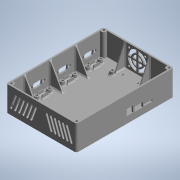
# Autodesk Inventor part: skr_case
Saved by Autodesk Inventor 2022 (Build 260153000, 153)
## iProperties
Part Number: skr_case
Material: Allgemein
Document SubType Name: Modellieren
Designer: Niclas
Appearance: Vorgabe
Author: Niclas
Autodesk Inventor part; units mm, degrees
ref_plane "YZ-Ebene" through (0, 0, 0) normal (1, 0, 0) x (0, 1, 0)
ref_plane "XZ-Ebene" through (0, 0, 0) normal (0, 1, 0) x (-1, 0, 0)
ref_plane "XY-Ebene" through (0, 0, 0) normal (0, 0, 1) x (1, 0, 0)
sketch "Skizze1" plane through (0, 0, 0) normal (0, 1, 0) x (-1, 0, 0)
  line L0 (0, 0) -> (-140, 0)
  line L1 (-140, 0) -> (-140, -194)
  line L2 (-140, -194) -> (0, -194)
  line L3 (0, -194) -> (0, 0)
  dimension "d0" = 194
  dimension "d1" = 140
  constraints: 8 end point, 2 parallel, 1 coincident, 1 horizontal, 1 perpendicular
  measures "d0" distance of L2.end L0.start
  measures "d1" distance of L0.start L0.end
extrude "Extrusion1" add sketch "Skizze1" along normal blind 5
sketch "Skizze2" plane through (0, 5, 0) normal (0, 1, 0) x (1, 0, 0)
  circle A0 centre (45, 28) radius 4
  circle A1 centre (45, 166) radius 4
  circle A2 centre (132, 28) radius 4
  circle A3 centre (132, 166) radius 4
  line L0 (140, 0) -> (140, 194) projected
  line L1 (140, 194) -> (0, 194) projected
  circle A4 centre (45, 28) radius 2.25
  circle A5 centre (132, 28) radius 2.25
  circle A6 centre (132, 166) radius 2.25
  circle A7 centre (45, 166) radius 2.25
  point P0 (0, 0)
  dimension "d4" = 138
  dimension "d5" = 138
  dimension "d6" = 87
  dimension "d7" = 87
  dimension "d8" = 8
  dimension "d9" = 8
  dimension "d10" = 8
  dimension "d11" = 8
  dimension "d12" = 8
  dimension "d13" = 8
  dimension "d14" = 28
  dimension "d15" = 28
  dimension "d16" = 4.5
  dimension "d17" = 4.5
  dimension "d18" = 4.5
  dimension "d19" = 4.5
  constraints: 8 centre point, 4 coincident
  measures "d4" distance of A3.centre A2.centre
  measures "d5" distance of A1.centre A0.centre
  measures "d6" distance of A2.centre A0.centre
  measures "d7" distance of A3.centre A1.centre
  measures "d8" distance from line of L0 A2.centre
  measures "d9" distance from line of L0 A3.centre
  measures "d10" diameter of A2
  measures "d11" diameter of A3
  measures "d12" diameter of A1
  measures "d13" diameter of A0
  measures "d14" distance from line of L1 A3.centre
  measures "d15" distance from line of L1 A1.centre
  measures "d16" diameter of A4
  measures "d17" diameter of A5
  measures "d18" diameter of A6
  measures "d19" diameter of A7
extrude "Extrusion2" add sketch "Skizze2" along normal blind 7
chamfer "Fase1" distance 2 angle 45 4 edges at (128, 5, -28) (41, 5, -28) (41, 5, -166) (128, 5, -166)
sketch "Skizze3" plane through (0, 5, 0) normal (0, 1, 0) x (1, 0, 0)
  line L0 (3, 3) -> (137, 3)
  line L1 (137, 3) -> (137, 191)
  line L2 (137, 191) -> (3, 191)
  line L3 (3, 191) -> (3, 3)
  line L4 (0, 194) -> (0, 0) projected
  line L5 (0, 0) -> (140, 0) projected
  line L6 (140, 0) -> (140, 194) projected
  line L7 (140, 194) -> (0, 194) projected
  line L8 (0, 0) -> (140, 0)
  line L9 (140, 0) -> (140, 194)
  line L10 (140, 194) -> (0, 194)
  line L11 (0, 194) -> (0, 0)
  dimension "d25" = 3
  dimension "d26" = 3
  dimension "d27" = 3
  dimension "d28" = 3
  constraints: 16 end point, 4 parallel, 2 horizontal, 2 perpendicular
  measures "d25" distance between parallel lines of L3 L4
  measures "d26" distance between parallel lines of L5 L0
  measures "d27" distance between parallel lines of L6 L1
  measures "d28" distance between parallel lines of L7 L2
extrude "Extrusion3" add sketch "Skizze3" along normal blind 45
sketch "Skizze4" plane through (140, 0, 0) normal (1, 0, 0) x (0, 0, -1)
  line L0 (99.85, 25.4) -> (112.85, 25.4)
  line L1 (112.85, 25.4) -> (112.85, 13.4)
  line L2 (112.85, 13.4) -> (99.85, 13.4)
  line L3 (99.85, 13.4) -> (99.85, 25.4)
  line L4 (0, 0) -> (194, 0) projected
  line L5 (194, 0) -> (194, 50) projected
  line L6 (115.9, 21.6) -> (132.4, 21.6)
  line L7 (132.4, 21.6) -> (132.4, 12.6)
  line L8 (132.4, 12.6) -> (115.9, 12.6)
  line L9 (115.9, 12.6) -> (115.9, 21.6)
  line L10 (134.15, 16.8) -> (151.15, 16.8)
  line L11 (151.15, 16.8) -> (151.15, 13.3)
  line L12 (151.15, 13.3) -> (134.15, 13.3)
  line L13 (134.15, 13.3) -> (134.15, 16.8)
  dimension "d31" = 12
  dimension "d32" = 13
  dimension "d33" = 13.4
  dimension "d34" = 81.15
  dimension "d37" = 9
  dimension "d38" = 16.5
  dimension "d39" = 61.6
  dimension "d40" = 12.6
  dimension "d41" = 17
  dimension "d42" = 3.5
  dimension "d43" = 42.85
  dimension "d44" = 13.3
  constraints: 24 end point, 6 parallel, 3 horizontal, 3 perpendicular
  measures "d31" distance of L0.end L1.end
  measures "d32" distance of L1.end L2.end
  measures "d33" distance between parallel lines of L4 L2
  measures "d34" distance between parallel lines of L5 L1
  measures "d37" distance of L6.end L7.end
  measures "d38" distance of L7.end L8.end
  measures "d39" distance between parallel lines of L5 L7
  measures "d40" distance between parallel lines of L4 L8
  measures "d41" distance of L10.start L10.end
  measures "d42" distance of L10.end L11.end
  measures "d43" distance between parallel lines of L5 L11
  measures "d44" distance between parallel lines of L4 L12
extrude "Extrusion4" cut sketch "Skizze4" against normal blind 40
sketch "Skizze5" plane through (0, 0, -194) normal (-1, 0, 0) x (0, 0, 1)
  line L0 (128.4836, 25) -> (140.5164, 25)
  line L1 (143.4832, 21.555) -> (142.8832, 17.555)
  line L2 (139.9164, 15) -> (129.0836, 15)
  line L3 (126.1168, 17.555) -> (125.5168, 21.555)
  arc A0 (128.4836, 25) -> (125.5168, 21.555) centre (128.4836, 22) ccw
  arc A1 (126.1168, 17.555) -> (129.0836, 15) centre (129.0836, 18) ccw
  arc A2 (139.9164, 15) -> (142.8832, 17.555) centre (139.9164, 18) ccw
  arc A3 (143.4832, 21.555) -> (140.5164, 25) centre (140.5164, 22) ccw
  circle A4 centre (122, 20) radius 2.75
  circle A5 centre (147, 20) radius 2.75
  line L4 (77.4836, 25) -> (89.5164, 25)
  line L5 (92.4832, 21.555) -> (91.8832, 17.555)
  line L6 (88.9164, 15) -> (78.0836, 15)
  line L7 (75.1168, 17.555) -> (74.5168, 21.555)
  arc A6 (77.4836, 25) -> (74.5168, 21.555) centre (77.4836, 22) ccw
  arc A7 (75.1168, 17.555) -> (78.0836, 15) centre (78.0836, 18) ccw
  arc A8 (88.9164, 15) -> (91.8832, 17.555) centre (88.9164, 18) ccw
  arc A9 (92.4832, 21.555) -> (89.5164, 25) centre (89.5164, 22) ccw
  circle A10 centre (71, 20) radius 2.75
  circle A11 centre (96, 20) radius 2.75
  line L8 (26.4836, 25) -> (38.5164, 25)
  line L9 (41.4832, 21.555) -> (40.8832, 17.555)
  line L10 (37.9164, 15) -> (27.0836, 15)
  line L11 (24.1168, 17.555) -> (23.5168, 21.555)
  arc A12 (26.4836, 25) -> (23.5168, 21.555) centre (26.4836, 22) ccw
  arc A13 (24.1168, 17.555) -> (27.0836, 15) centre (27.0836, 18) ccw
  arc A14 (37.9164, 15) -> (40.8832, 17.555) centre (37.9164, 18) ccw
  arc A15 (41.4832, 21.555) -> (38.5164, 25) centre (38.5164, 22) ccw
  circle A16 centre (20, 20) radius 2.75
  circle A17 centre (45, 20) radius 2.75
  line L12 (0, 50) -> (194, 50) projected
  line L13 (0, 0) -> (0, 50) projected
  circle A18 centre (172.5, 20) radius 4
  line L14 (0, 0) -> (194, 0) projected
  point P0 (125, 25)
  point P1 (144, 25)
  point P2 (142.5, 15)
  point P3 (126.5, 15)
  point P4 (74, 25)
  point P5 (93, 25)
  point P6 (91.5, 15)
  point P7 (75.5, 15)
  point P8 (23, 25)
  point P9 (42, 25)
  point P10 (40.5, 15)
  point P11 (24.5, 15)
  dimension "d45" = 19
  dimension "d46" = 16
  dimension "d47" = 10
  dimension "d48" = 1.5
  dimension "d49" = 3
  dimension "d50" = 25
  dimension "d51" = 5.5
  dimension "d52" = 5.5
  dimension "d53" = 5
  dimension "d54" = 5
  dimension "d55" = 4.5
  dimension "d56" = 19
  dimension "d57" = 16
  dimension "d58" = 10
  dimension "d59" = 1.5
  dimension "d60" = 3
  dimension "d61" = 25
  dimension "d62" = 5.5
  dimension "d63" = 5.5
  dimension "d64" = 5
  dimension "d65" = 5
  dimension "d66" = 4.5
  dimension "d67" = 19
  dimension "d68" = 16
  dimension "d69" = 10
  dimension "d70" = 1.5
  dimension "d71" = 3
  dimension "d72" = 25
  dimension "d73" = 5.5
  dimension "d74" = 5.5
  dimension "d75" = 5
  dimension "d76" = 5
  dimension "d77" = 4.5
  dimension "d142" = 20
  dimension "d143" = 26
  dimension "d144" = 26
  dimension "d145" = 8
  dimension "d146" = 25.5
  dimension "d147" = 0
  dimension "d267" = 20
  dimension "d268" = 20
  dimension "d269" = 20
  constraints: 24 end point, 24 point on circle, 24 point on line, 24 tangent, 19 centre point, 9 equal radius, 3 horizontal, 3 parallel
  measures "d45" distance of point (125, 25) point (144, 25)
  measures "d46" distance of point (142.5, 15) point (126.5, 15)
  measures "d47" vertical distance of point (126.5, 15) point (125, 25)
  measures "d48" horizontal distance of point (125, 25) point (126.5, 15)
  measures "d49" radius of A0
  measures "d50" distance of A5.centre A4.centre
  measures "d51" diameter of A5
  measures "d52" diameter of A4
  measures "d53" vertical distance of point (142.5, 15) A5.centre
  measures "d54" vertical distance of point (126.5, 15) A4.centre
  measures "d55" horizontal distance of point (142.5, 15) A5.centre
  measures "d56" distance of point (74, 25) point (93, 25)
  measures "d57" distance of point (91.5, 15) point (75.5, 15)
  measures "d58" vertical distance of point (75.5, 15) point (74, 25)
  measures "d59" horizontal distance of point (74, 25) point (75.5, 15)
  measures "d60" radius of A6
  measures "d61" distance of A11.centre A10.centre
  measures "d62" diameter of A11
  measures "d63" diameter of A10
  measures "d64" vertical distance of point (91.5, 15) A11.centre
  measures "d65" vertical distance of point (75.5, 15) A10.centre
  measures "d66" horizontal distance of point (91.5, 15) A11.centre
  measures "d67" distance of point (23, 25) point (42, 25)
  measures "d68" distance of point (40.5, 15) point (24.5, 15)
  measures "d69" vertical distance of point (24.5, 15) point (23, 25)
  measures "d70" horizontal distance of point (23, 25) point (24.5, 15)
  measures "d71" radius of A12
  measures "d72" distance of A17.centre A16.centre
  measures "d73" diameter of A17
  measures "d74" diameter of A16
  measures "d75" vertical distance of point (40.5, 15) A17.centre
  measures "d76" vertical distance of point (24.5, 15) A16.centre
  measures "d77" horizontal distance of point (40.5, 15) A17.centre
  measures "d142" distance from line of L13 A16.centre
  measures "d143" distance of A17.centre A10.centre
  measures "d144" distance of A11.centre A4.centre
  measures "d145" diameter of A18
  measures "d146" distance of A5.centre A18.centre
  measures "d147" vertical distance of A5.centre A18.centre
  measures "d267" distance from line of L14 A16.centre
  measures "d268" distance from line of L14 A10.centre
  measures "d269" distance from line of L14 A4.centre
extrude "Extrusion5" cut sketch "Skizze5" against normal blind 40
sketch "Skizze6" plane through (0, 5, 0) normal (0, 1, 0) x (1, 0, 0)
  circle A0 centre (13.5, 149) radius 4
  circle A1 centre (13.5, 174) radius 4
  circle A2 centre (13.5, 149) radius 2.25
  circle A3 centre (13.5, 174) radius 2.25
  line L0 (140, 194) -> (0, 194) projected
  line L1 (0, 194) -> (0, 0) projected
  line L2 (8.5, 155.5) -> (9.5, 155.5)
  line L3 (9.5, 155.5) -> (9.5, 167.5)
  line L4 (9.5, 167.5) -> (8.5, 167.5)
  line L5 (8.5, 167.5) -> (8.5, 155.5)
  line L6 (17.5, 155.5) -> (18.5, 155.5)
  line L7 (18.5, 155.5) -> (18.5, 167.5)
  line L8 (18.5, 167.5) -> (17.5, 167.5)
  line L9 (17.5, 167.5) -> (17.5, 155.5)
  circle A4 centre (13.5, 98) radius 4
  circle A5 centre (13.5, 123) radius 4
  circle A6 centre (13.5, 98) radius 2.25
  circle A7 centre (13.5, 123) radius 2
  line L10 (8.5, 104.5) -> (9.5, 104.5)
  line L11 (9.5, 104.5) -> (9.5, 116.5)
  line L12 (9.5, 116.5) -> (8.5, 116.5)
  line L13 (8.5, 116.5) -> (8.5, 104.5)
  line L14 (17.5, 104.5) -> (18.5, 104.5)
  line L15 (18.5, 104.5) -> (18.5, 116.5)
  line L16 (18.5, 116.5) -> (17.5, 116.5)
  line L17 (17.5, 116.5) -> (17.5, 104.5)
  line L18 (17.5, 53.5) -> (18.5, 53.5)
  line L19 (18.5, 53.5) -> (18.5, 65.5)
  line L20 (17.5, 65.5) -> (17.5, 53.5)
  line L21 (8.5, 53.5) -> (9.5, 53.5)
  line L22 (9.5, 53.5) -> (9.5, 65.5)
  line L23 (8.5, 65.5) -> (8.5, 53.5)
  circle A8 centre (13.5, 47) radius 2.25
  circle A9 centre (13.5, 47) radius 4
  circle A10 centre (13.5, 72) radius 4
  circle A11 centre (13.5, 72) radius 2.25
  line L24 (9.5, 65.5) -> (8.5, 65.5)
  line L25 (18.5, 65.5) -> (17.5, 65.5)
  line L26 (3, 3) -> (3, 191) projected
  dimension "d86" = 8
  dimension "d87" = 8
  dimension "d88" = 25
  dimension "d89" = 4.5
  dimension "d90" = 4.5
  dimension "d91" = 20
  dimension "d94" = 1
  dimension "d95" = 12
  dimension "d96" = 12
  dimension "d97" = 1
  dimension "d98" = 4
  dimension "d99" = 4
  dimension "d100" = 6.5
  dimension "d101" = 8
  dimension "d102" = 8
  dimension "d103" = 25
  dimension "d104" = 4.5
  dimension "d105" = 4
  dimension "d106" = 1
  dimension "d107" = 12
  dimension "d108" = 12
  dimension "d109" = 1
  dimension "d110" = 4
  dimension "d111" = 4
  dimension "d112" = 6.5
  dimension "d113" = 26
  dimension "d116" = 8
  dimension "d117" = 8
  dimension "d118" = 25
  dimension "d119" = 4.5
  dimension "d120" = 4.5
  dimension "d121" = 1
  dimension "d122" = 12
  dimension "d123" = 12
  dimension "d124" = 1
  dimension "d125" = 4
  dimension "d126" = 4
  dimension "d127" = 6.5
  dimension "d128" = 26
  dimension "d131" = 10.5
  dimension "d132" = 10.5
  dimension "d133" = 10.5
  dimension "d134" = 10.5
  dimension "d135" = 10.5
  dimension "d136" = 10.5
  constraints: 48 end point, 12 centre point, 12 parallel, 6 coincident, 6 horizontal, 6 perpendicular, 3 point on line
  measures "d86" diameter of A1
  measures "d87" diameter of A0
  measures "d88" distance of A1.centre A0.centre
  measures "d89" diameter of A2
  measures "d90" diameter of A3
  measures "d91" distance from line of L0 A1.centre
  measures "d94" distance of L2.start L2.end
  measures "d95" distance of L4.end L2.start
  measures "d96" distance of L8.end L6.start
  measures "d97" distance of L6.start L6.end
  measures "d98" distance from line of L9 A0.centre
  measures "d99" distance from line of L3 A0.centre
  measures "d100" vertical distance of A0.centre L2.end
  measures "d101" diameter of A5
  measures "d102" diameter of A4
  measures "d103" distance of A5.centre A4.centre
  measures "d104" diameter of A6
  measures "d105" diameter of A7
  measures "d106" distance of L10.start L10.end
  measures "d107" distance of L13.start L10.start
  measures "d108" distance of L17.start L14.start
  measures "d109" distance of L14.start L14.end
  measures "d110" distance from line of L17 A4.centre
  measures "d111" distance from line of L11 A4.centre
  measures "d112" vertical distance of A4.centre L10.end
  measures "d113" distance of A7.centre A0.centre
  measures "d116" diameter of A10
  measures "d117" diameter of A9
  measures "d118" distance of A10.centre A9.centre
  measures "d119" diameter of A8
  measures "d120" diameter of A11
  measures "d121" distance of L21.start L22.start
  measures "d122" distance of L24.end L21.start
  measures "d123" distance of L25.end L18.start
  measures "d124" distance of L18.start L19.start
  measures "d125" distance from line of L20 A9.centre
  measures "d126" distance from line of L22 A9.centre
  measures "d127" vertical distance of A9.centre L22.start
  measures "d128" distance of A4.centre A11.centre
  measures "d131" distance from line of L26 A9.centre
  measures "d132" distance from line of L26 A11.centre
  measures "d133" distance from line of L26 A6.centre
  measures "d134" distance from line of L26 A5.centre
  measures "d135" distance from line of L26 A0.centre
  measures "d136" distance from line of L26 A1.centre
extrude "Extrusion6" add sketch "Skizze6" along normal blind 7.5
chamfer "Fase2" distance 2 angle 45 30 edges at (9.5, 5, -47) (9.5, 5, -72) (9.5, 5, -98) (9.5, 5, -123) (9.5, 5, -149) (9.5, 5, -174) (18.5, 5, -161.5) (18.5, 5, -110.5) (18.5, 5, -59.5) (9.5, 5, -110.5) (9.5, 5, -161.5) (9.5, 5, -59.5) (18, 5, -104.5) (18, 5, -53.5) (18, 5, -155.5) (9, 5, -53.5) (9, 5, -104.5) (9, 5, -155.5) (18, 5, -65.5) (18, 5, -116.5) (18, 5, -167.5) (9, 5, -167.5) (9, 5, -116.5) (9, 5, -65.5) (8.5, 5, -161.5) (8.5, 5, -110.5) (8.5, 5, -59.5) (17.5, 5, -59.5) (17.5, 5, -110.5) (17.5, 5, -161.5)
sketch "Skizze7" plane through (3, 5, -3) normal (1, 0, 0) x (0, 0, -1)
  line L0 (132, 0) -> (134, 0)
  line L1 (134, 0) -> (134, 45)
  line L2 (134, 45) -> (132, 45)
  line L3 (132, 45) -> (132, 0)
  circle A0 centre (120, 15) radius 2.75 projected
  line L4 (81, 0) -> (83, 0)
  line L5 (83, 0) -> (83, 45)
  line L6 (83, 45) -> (81, 45)
  line L7 (81, 45) -> (81, 0)
  circle A1 centre (69, 15) radius 2.75 projected
  line L8 (32, 0) -> (30, 0)
  line L9 (30, 0) -> (30, 45)
  line L10 (30, 45) -> (32, 45)
  line L11 (32, 45) -> (32, 0)
  circle A2 centre (18.5, 15) radius 4 projected
  circle A3 centre (171, 15) radius 2.75 projected
  circle A4 centre (146, 15) radius 2.75 projected
  circle A5 centre (95, 15) radius 2.75 projected
  circle A6 centre (44, 15) radius 2.75 projected
  line L12 (0, 45) -> (188, 45) projected
  line L13 (188, 0) -> (0, 0) projected
  point P0 (-3, -5)
  dimension "d149" = 2
  dimension "d151" = 2
  dimension "d153" = 2
  dimension "d368" = 12
  dimension "d369" = 12
  dimension "d376" = 12
  constraints: 24 end point, 6 parallel, 6 point on line, 3 horizontal, 3 perpendicular
  measures "d149" distance between parallel lines of L1 L3
  measures "d151" distance of L6.end L5.end
  measures "d153" distance of L9.end L10.end
  measures "d368" distance from line of L1 A4.centre
  measures "d369" distance from line of L5 A5.centre
  measures "d376" distance from line of L11 A6.centre
extrude "Extrusion7" add sketch "Skizze7" along normal blind 25 contours L3 L2 L1 L0 | L4 L7 L6 L5 | L8 L9 L10 L11
sketch "Skizze9" plane through (140, 0, -194) normal (0, 0, -1) x (-1, 0, 0)
  circle A0 centre (70, 27.5) radius 19
  line L0 (140, 0) -> (140, 50) projected
  line L1 (0, 50) -> (140, 50) projected
  circle A1 centre (70, 27.5) radius 12.5
  circle A2 centre (70, 27.5) radius 10
  line L2 (90, 29) -> (50, 29)
  line L3 (50, 29) -> (50, 26)
  line L4 (50, 26) -> (90, 26)
  line L5 (90, 26) -> (90, 29)
  line L6 (68.5, 47.5) -> (71.5, 47.5)
  line L7 (71.5, 47.5) -> (71.5, 7.5)
  line L8 (71.5, 7.5) -> (68.5, 7.5)
  line L9 (68.5, 7.5) -> (68.5, 47.5)
  circle A3 centre (86, 43.5) radius 2
  circle A4 centre (86, 11.5) radius 2
  circle A5 centre (54, 11.5) radius 2
  circle A6 centre (54, 43.5) radius 2
  point P0 (68.5, 29)
  point P1 (68.5, 37.3869)
  point P2 (60.1131, 29)
  point P3 (68.5, 17.6131)
  point P4 (68.5, 26)
  point P5 (60.1131, 26)
  point P6 (71.5, 26)
  point P7 (71.5, 17.6131)
  point P8 (79.8869, 26)
  point P9 (71.5, 37.3869)
  point P10 (71.5, 29)
  point P11 (79.8869, 29)
  point P12 (71.5, 46.4407)
  point P13 (71.5, 39.9097)
  point P14 (82.4097, 29)
  point P15 (88.9407, 29)
  point P16 (71.5, 15.0903)
  point P17 (71.5, 8.5593)
  point P18 (88.9407, 26)
  point P19 (82.4097, 26)
  point P20 (68.5, 8.5593)
  point P21 (68.5, 15.0903)
  point P22 (57.5903, 26)
  point P23 (51.0593, 26)
  point P24 (68.5, 39.9097)
  point P25 (68.5, 46.4407)
  point P26 (51.0593, 29)
  point P27 (57.5903, 29)
  dimension "d163" = 38
  dimension "d164" = 70
  dimension "d165" = 22.5
  dimension "d166" = 25
  dimension "d167" = 20
  dimension "d168" = 3
  dimension "d169" = 1.5
  dimension "d170" = 20
  dimension "d171" = 20
  dimension "d172" = 3
  dimension "d173" = 20
  dimension "d174" = 20
  dimension "d175" = 1.5
  dimension "d178" = 4
  dimension "d179" = 4
  dimension "d180" = 4
  dimension "d181" = 4
  dimension "d182" = 32
  dimension "d183" = 32
  dimension "d184" = 32
  dimension "d185" = 32
  dimension "d186" = 16
  dimension "d187" = 16
  dimension "d188" = 16
  dimension "d189" = 16
  constraints: 16 end point, 7 centre point, 4 parallel, 2 coincident, 2 horizontal, 2 perpendicular
  measures "d163" diameter of A0
  measures "d164" distance from line of L0 A0.centre
  measures "d165" distance from line of A0.centre L1
  measures "d166" diameter of A1
  measures "d167" diameter of A2
  measures "d168" distance between parallel lines of L4 L2
  measures "d169" distance from line of A0.centre L2
  measures "d170" distance from line of A0.centre L5
  measures "d171" distance from line of A0.centre L3
  measures "d172" distance between parallel lines of L7 L9
  measures "d173" distance from line of A0.centre L6
  measures "d174" distance from line of A0.centre L8
  measures "d175" distance from line of A0.centre L7
  measures "d178" diameter of A3
  measures "d179" diameter of A5
  measures "d180" diameter of A6
  measures "d181" diameter of A4
  measures "d182" distance of A3.centre A6.centre
  measures "d183" distance of A5.centre A4.centre
  measures "d184" distance of A4.centre A3.centre
  measures "d185" distance of A5.centre A6.centre
  measures "d186" horizontal distance of A5.centre A0.centre
  measures "d187" horizontal distance of A0.centre A3.centre
  measures "d188" horizontal distance of A0.centre A4.centre
  measures "d189" horizontal distance of A0.centre A6.centre
extrude "Extrusion9" cut sketch "Skizze9" against normal blind 5 contours L2 A1 L7 A0 | A0 L7 A1 L4 | L9 A1 L2 A0 | L2 L7 A2 | A0 L4 A1 L9 | A2 L7 L4 | L9 L2 A2 | A2 L4 L9 | A3 | A4 | A5 | A6
sketch "Skizze10" plane through (3, 5, -191) normal (0, 0, 1) x (1, 0, 0)
  line L0 (90.5, 0) -> (92.5, 0)
  line L1 (92.5, 0) -> (92.5, 45)
  line L2 (92.5, 45) -> (90.5, 45)
  line L3 (90.5, 45) -> (90.5, 0)
  line L4 (134, 0) -> (0, 0) projected
  line L5 (0, 45) -> (134, 45) projected
  line L6 (43.5, 0) -> (41.5, 0)
  line L7 (41.5, 0) -> (41.5, 45)
  line L8 (41.5, 45) -> (43.5, 45)
  line L9 (43.5, 45) -> (43.5, 0)
  line L10 (65.5, 32.3869) -> (65.5, 24) projected
  line L11 (68.5, 12.6131) -> (68.5, 21) projected
  point P0 (-3, -5)
  point P1 (41.5, 0)
  dimension "d190" = 2
  dimension "d191" = 2
  dimension "d192" = 22
  dimension "d193" = 22
  dimension "d196" = 0
  constraints: 16 end point, 4 parallel, 3 point on line, 2 horizontal, 2 perpendicular
  measures "d190" distance of L1.end L2.end
  measures "d191" distance between parallel lines of L9 L7
  measures "d192" distance between parallel lines of L10 L9
  measures "d193" distance between parallel lines of L11 L3
  measures "d196" distance between parallel lines of L2 L5
extrude "Extrusion10" add sketch "Skizze10" along normal blind 20 contours L3 L2 L1 L0 | L4 L7 L5 L9
sketch "Skizze12" plane through (95.5, 5, -191) normal (1, 0, 0) x (0, 0, -1)
  line L0 (0, 45) -> (-20, 45) projected
  line L1 (-20, 0) -> (0, 45)
  line L2 (0, 45) -> (-20, 45)
  line L3 (-20, 45) -> (-20, 0)
  point P0 (-191, -5)
  constraints: 6 end point, 1 perpendicular
extrude "Extrusion11" cut sketch "Skizze12" against normal blind 52
sketch "Skizze13" plane through (0, 0, 0) normal (0, 0, 1) x (1, 0, 0)
  line L0 (0, 0) -> (0, 50) projected
  line L1 (17.0131, 37.884) -> (8.1206, 13.452)
  line L2 (17.6972, 39.7634) -> (43.6972, 39.7634) construction
  line L3 (9.316, 10.8886) -> (9.316, 10.8886)
  line L4 (11.8794, 12.084) -> (20.7719, 36.516)
  line L5 (19.5766, 39.0794) -> (19.5766, 39.0794)
  arc A0 (19.5766, 39.0794) -> (17.0131, 37.884) centre (18.8925, 37.2) ccw
  arc A1 (20.7719, 36.516) -> (19.5766, 39.0794) centre (18.8925, 37.2) ccw
  arc A2 (9.316, 10.8886) -> (11.8794, 12.084) centre (10, 12.768) ccw
  arc A3 (8.1206, 13.452) -> (9.316, 10.8886) centre (10, 12.768) ccw
  line L6 (0, 50) -> (140, 50) projected
  line L7 (25.0131, 37.884) -> (16.1206, 13.452)
  line L8 (17.316, 10.8886) -> (17.316, 10.8886)
  line L9 (19.8794, 12.084) -> (28.7719, 36.516)
  line L10 (27.5766, 39.0794) -> (27.5766, 39.0794)
  arc A4 (27.5766, 39.0794) -> (25.0131, 37.884) centre (26.8925, 37.2) ccw
  arc A5 (28.7719, 36.516) -> (27.5766, 39.0794) centre (26.8925, 37.2) ccw
  arc A6 (17.316, 10.8886) -> (19.8794, 12.084) centre (18, 12.768) ccw
  arc A7 (16.1206, 13.452) -> (17.316, 10.8886) centre (18, 12.768) ccw
  line L11 (33.0131, 37.884) -> (24.1206, 13.452)
  line L12 (25.316, 10.8886) -> (25.316, 10.8886)
  line L13 (27.8794, 12.084) -> (36.7719, 36.516)
  line L14 (35.5766, 39.0794) -> (35.5766, 39.0794)
  arc A8 (35.5766, 39.0794) -> (33.0131, 37.884) centre (34.8925, 37.2) ccw
  arc A9 (36.7719, 36.516) -> (35.5766, 39.0794) centre (34.8925, 37.2) ccw
  arc A10 (25.316, 10.8886) -> (27.8794, 12.084) centre (26, 12.768) ccw
  arc A11 (24.1206, 13.452) -> (25.316, 10.8886) centre (26, 12.768) ccw
  line L15 (41.0131, 37.884) -> (32.1206, 13.452)
  line L16 (33.316, 10.8886) -> (33.316, 10.8886)
  line L17 (35.8794, 12.084) -> (44.7719, 36.516)
  line L18 (43.5766, 39.0794) -> (43.5766, 39.0794)
  arc A12 (43.5766, 39.0794) -> (41.0131, 37.884) centre (42.8925, 37.2) ccw
  arc A13 (44.7719, 36.516) -> (43.5766, 39.0794) centre (42.8925, 37.2) ccw
  arc A14 (33.316, 10.8886) -> (35.8794, 12.084) centre (34, 12.768) ccw
  arc A15 (32.1206, 13.452) -> (33.316, 10.8886) centre (34, 12.768) ccw
  line L19 (49.0131, 37.884) -> (40.1206, 13.452)
  line L20 (41.316, 10.8886) -> (41.316, 10.8886)
  line L21 (43.8794, 12.084) -> (52.7719, 36.516)
  line L22 (51.5766, 39.0794) -> (51.5766, 39.0794)
  arc A16 (51.5766, 39.0794) -> (49.0131, 37.884) centre (50.8925, 37.2) ccw
  arc A17 (52.7719, 36.516) -> (51.5766, 39.0794) centre (50.8925, 37.2) ccw
  arc A18 (41.316, 10.8886) -> (43.8794, 12.084) centre (42, 12.768) ccw
  arc A19 (40.1206, 13.452) -> (41.316, 10.8886) centre (42, 12.768) ccw
  line L23 (57.0131, 37.884) -> (48.1206, 13.452)
  line L24 (49.316, 10.8886) -> (49.316, 10.8886)
  line L25 (51.8794, 12.084) -> (60.7719, 36.516)
  line L26 (59.5766, 39.0794) -> (59.5766, 39.0794)
  arc A20 (59.5766, 39.0794) -> (57.0131, 37.884) centre (58.8925, 37.2) ccw
  arc A21 (60.7719, 36.516) -> (59.5766, 39.0794) centre (58.8925, 37.2) ccw
  arc A22 (49.316, 10.8886) -> (51.8794, 12.084) centre (50, 12.768) ccw
  arc A23 (48.1206, 13.452) -> (49.316, 10.8886) centre (50, 12.768) ccw
  line L27 (137, 50) -> (3, 50) projected
  line L28 (70, 50) -> (70, 0)
  line L29 (0, 0) -> (140, 0) projected
  line L30 (140, 0) -> (140, 50) projected
  line L31 (122.9869, 37.884) -> (131.8794, 13.452)
  line L32 (122.3028, 39.7634) -> (96.3028, 39.7634) construction
  line L33 (130.684, 10.8886) -> (130.684, 10.8886)
  line L34 (128.1206, 12.084) -> (119.2281, 36.516)
  line L35 (120.4234, 39.0794) -> (120.4234, 39.0794)
  arc A24 (122.9869, 37.884) -> (120.4234, 39.0794) centre (121.1075, 37.2) ccw
  arc A25 (120.4234, 39.0794) -> (119.2281, 36.516) centre (121.1075, 37.2) ccw
  arc A26 (128.1206, 12.084) -> (130.684, 10.8886) centre (130, 12.768) ccw
  arc A27 (130.684, 10.8886) -> (131.8794, 13.452) centre (130, 12.768) ccw
  line L36 (114.9869, 37.884) -> (123.8794, 13.452)
  line L37 (120.1206, 12.084) -> (111.2281, 36.516)
  line L38 (112.4234, 39.0794) -> (112.4234, 39.0794)
  arc A28 (114.9869, 37.884) -> (112.4234, 39.0794) centre (113.1075, 37.2) ccw
  arc A29 (112.4234, 39.0794) -> (111.2281, 36.516) centre (113.1075, 37.2) ccw
  arc A30 (122.684, 10.8886) -> (123.8794, 13.452) centre (122, 12.768) ccw
  arc A31 (120.1206, 12.084) -> (122.684, 10.8886) centre (122, 12.768) ccw
  line L39 (122.684, 10.8886) -> (122.684, 10.8886)
  line L40 (106.9869, 37.884) -> (115.8794, 13.452)
  line L41 (112.1206, 12.084) -> (103.2281, 36.516)
  line L42 (104.4234, 39.0794) -> (104.4234, 39.0794)
  arc A32 (106.9869, 37.884) -> (104.4234, 39.0794) centre (105.1075, 37.2) ccw
  arc A33 (104.4234, 39.0794) -> (103.2281, 36.516) centre (105.1075, 37.2) ccw
  arc A34 (114.684, 10.8886) -> (115.8794, 13.452) centre (114, 12.768) ccw
  arc A35 (112.1206, 12.084) -> (114.684, 10.8886) centre (114, 12.768) ccw
  line L43 (114.684, 10.8886) -> (114.684, 10.8886)
  line L44 (98.9869, 37.884) -> (107.8794, 13.452)
  line L45 (104.1206, 12.084) -> (95.2281, 36.516)
  line L46 (96.4234, 39.0794) -> (96.4234, 39.0794)
  arc A36 (98.9869, 37.884) -> (96.4234, 39.0794) centre (97.1075, 37.2) ccw
  arc A37 (96.4234, 39.0794) -> (95.2281, 36.516) centre (97.1075, 37.2) ccw
  arc A38 (106.684, 10.8886) -> (107.8794, 13.452) centre (106, 12.768) ccw
  arc A39 (104.1206, 12.084) -> (106.684, 10.8886) centre (106, 12.768) ccw
  line L47 (106.684, 10.8886) -> (106.684, 10.8886)
  line L48 (90.9869, 37.884) -> (99.8794, 13.452)
  line L49 (96.1206, 12.084) -> (87.2281, 36.516)
  line L50 (88.4234, 39.0794) -> (88.4234, 39.0794)
  arc A40 (90.9869, 37.884) -> (88.4234, 39.0794) centre (89.1075, 37.2) ccw
  arc A41 (88.4234, 39.0794) -> (87.2281, 36.516) centre (89.1075, 37.2) ccw
  arc A42 (98.684, 10.8886) -> (99.8794, 13.452) centre (98, 12.768) ccw
  arc A43 (96.1206, 12.084) -> (98.684, 10.8886) centre (98, 12.768) ccw
  line L51 (98.684, 10.8886) -> (98.684, 10.8886)
  line L52 (82.9869, 37.884) -> (91.8794, 13.452)
  line L53 (88.1206, 12.084) -> (79.2281, 36.516)
  line L54 (80.4234, 39.0794) -> (80.4234, 39.0794)
  arc A44 (82.9869, 37.884) -> (80.4234, 39.0794) centre (81.1075, 37.2) ccw
  arc A45 (80.4234, 39.0794) -> (79.2281, 36.516) centre (81.1075, 37.2) ccw
  arc A46 (90.684, 10.8886) -> (91.8794, 13.452) centre (90, 12.768) ccw
  arc A47 (88.1206, 12.084) -> (90.684, 10.8886) centre (90, 12.768) ccw
  line L55 (90.684, 10.8886) -> (90.684, 10.8886)
  point P0 (7.4366, 11.5726)
  point P1 (11.1953, 10.2046)
  point P2 (25.6972, 39.7634)
  point P3 (15.4366, 11.5726)
  point P4 (19.1953, 10.2046)
  point P5 (33.6972, 39.7634)
  point P6 (23.4366, 11.5726)
  point P7 (27.1953, 10.2046)
  point P8 (41.6972, 39.7634)
  point P9 (31.4366, 11.5726)
  point P10 (35.1953, 10.2046)
  point P11 (49.6972, 39.7634)
  point P12 (39.4366, 11.5726)
  point P13 (43.1953, 10.2046)
  point P14 (57.6972, 39.7634)
  point P15 (47.4366, 11.5726)
  point P16 (51.1953, 10.2046)
  point P17 (132.5634, 11.5726)
  point P18 (128.8047, 10.2046)
  point P19 (114.3028, 39.7634)
  point P20 (124.5634, 11.5726)
  point P21 (120.8047, 10.2046)
  point P22 (106.3028, 39.7634)
  point P23 (116.5634, 11.5726)
  point P24 (112.8047, 10.2046)
  point P25 (98.3028, 39.7634)
  point P26 (108.5634, 11.5726)
  point P27 (104.8047, 10.2046)
  point P28 (90.3028, 39.7634)
  point P29 (100.5634, 11.5726)
  point P30 (96.8047, 10.2046)
  point P31 (82.3028, 39.7634)
  point P32 (92.5634, 11.5726)
  point P33 (88.8047, 10.2046)
  point P34 (96.4234, 39.0794)
  point P35 (106.684, 10.8886)
  point P36 (90.684, 10.8886)
  point P37 (49.316, 10.8886)
  point P38 (33.316, 10.8886)
  point P39 (43.5766, 39.0794)
  point P40 (17.316, 10.8886)
  point P41 (9.316, 10.8886)
  point P42 (19.5766, 39.0794)
  dimension "d203" = 30
  dimension "d204" = 110
  dimension "d205" = 4
  dimension "d206" = 2
  dimension "d207" = 12.8
  dimension "d208" = 10
  dimension "d209" = 30
  dimension "d210" = 4
  dimension "d211" = 2
  dimension "d212" = 30
  dimension "d213" = 4
  dimension "d214" = 2
  dimension "d215" = 30
  dimension "d216" = 4
  dimension "d217" = 2
  dimension "d218" = 30
  dimension "d219" = 4
  dimension "d220" = 2
  dimension "d221" = 30
  dimension "d222" = 4
  dimension "d223" = 2
  dimension "d242" = 8
  dimension "d243" = 8
  dimension "d244" = 8
  dimension "d245" = 8
  dimension "d246" = 8
  dimension "d247" = 12.8
  dimension "d248" = 12.8
  dimension "d249" = 8
  dimension "d250" = 8
  dimension "d251" = 8
  dimension "d252" = 8
  dimension "d253" = 8
  dimension "d254" = 12.8
  dimension "d255" = 12.8
  dimension "d256" = 12.8
  dimension "d257" = 70
  constraints: 102 end point, 96 point on circle, 91 symmetric about line, 72 point on line, 48 centre point, 48 tangent, 18 equal radius, 18 perpendicular, 2 midpoint, 1 equal length, 1 horizontal, 1 vertical, 24 other
  measures "d203" distance of L2.start point (7.437, 11.573)
  measures "d204" angle of L1 L2
  measures "d205" distance of point (7.437, 11.573) point (11.195, 10.205)
  measures "d206" radius of A0
  measures "d207" distance from line of L6 A0.centre
  measures "d208" distance from line of L0 A3.centre
  measures "d209" distance of point (25.697, 39.763) point (15.437, 11.573)
  measures "d210" distance of point (15.437, 11.573) point (19.195, 10.205)
  measures "d211" radius of A4
  measures "d212" distance of point (33.697, 39.763) point (23.437, 11.573)
  measures "d213" distance of point (23.437, 11.573) point (27.195, 10.205)
  measures "d214" radius of A8
  measures "d215" distance of point (41.697, 39.763) point (31.437, 11.573)
  measures "d216" distance of point (31.437, 11.573) point (35.195, 10.205)
  measures "d217" radius of A12
  measures "d218" distance of point (49.697, 39.763) point (39.437, 11.573)
  measures "d219" distance of point (39.437, 11.573) point (43.195, 10.205)
  measures "d220" radius of A16
  measures "d221" distance of point (57.697, 39.763) point (47.437, 11.573)
  measures "d222" distance of point (47.437, 11.573) point (51.195, 10.205)
  measures "d223" radius of A20
  measures "d242" distance of A6.centre A2.centre
  measures "d243" distance of A10.centre A7.centre
  measures "d244" distance of A14.centre A11.centre
  measures "d245" distance of A15.centre A18.centre
  measures "d246" distance of A22.centre A18.centre
  measures "d247" distance from line of L6 A4.centre
  measures "d248" distance from line of L6 A8.centre
  measures "d249" distance of A1.centre A4.centre
  measures "d250" distance of A4.centre A9.centre
  measures "d251" distance of A8.centre A12.centre
  measures "d252" distance of A13.centre A17.centre
  measures "d253" distance of A20.centre A16.centre
  measures "d254" distance from line of L6 A13.centre
  measures "d255" distance from line of L6 A16.centre
  measures "d256" distance from line of L6 A21.centre
  measures "d257" distance between parallel lines of L30 L28
extrude "Extrusion12" cut sketch "Skizze13" against normal blind 5 contours A0 A1 L4 A2 A3 L1 | A4 A5 L9 A6 A7 L7 | A8 A9 L13 A10 A11 L11 | A12 A13 L17 A14 A15 L15 | A16 A17 L21 A18 A19 L19 | A20 A21 L25 A22 A23 L23 | L31 A27 A26 L34 A25 A24 | L36 A30 A31 L37 A29 A28 | L40 A34 A35 L41 A33 A32 | L44 A38 A39 L45 A37 A36 | L48 A42 A43 L49 A41 A40 | L52 A46 A47 L53 A45 A44
sketch "Skizze14" plane through (137, 5, -3) normal (0, 0, -1) x (-1, 0, 0)
  line L0 (0, 45) -> (134, 45) projected
  line L1 (69, 0) -> (65, 0)
  line L2 (65, 0) -> (65, 45)
  line L3 (65, 45) -> (69, 45)
  line L4 (69, 45) -> (69, 0)
  line L5 (134, 0) -> (134, 45) projected
  line L6 (134, 0) -> (0, 0) projected
  point P0 (137, -5)
  dimension "d260" = 4
  dimension "d261" = 65
  dimension "d262" = 0
  constraints: 8 end point, 2 parallel, 1 horizontal, 1 perpendicular, 1 point on line
  measures "d260" distance between parallel lines of L2 L4
  measures "d261" distance between parallel lines of L5 L4
  measures "d262" distance between parallel lines of L6 L1
extrude "Extrusion13" add sketch "Skizze14" along normal blind 20 contours L0 L4 L1 L2
sketch "Skizze15" plane through (72, 5, -3) normal (1, 0, 0) x (0, 0, -1)
  line L0 (0, 45) -> (20, 45) projected
  line L1 (20, 45) -> (20, 0) projected
  line L2 (0, 45) -> (20, 0)
  line L3 (0, 0) -> (0, 45) projected
  line L4 (20, 0) -> (0, 0)
  line L5 (0, 0) -> (0, 45)
  line L6 (0, 45) -> (20, 45)
  line L7 (20, 45) -> (20, 0)
  point P0 (-3, -5)
  constraints: 10 end point, 2 collinear, 1 perpendicular
extrude "Extrusion14" cut sketch "Skizze15" against normal blind 5 contours L0 L1 L2
sketch "Skizze16" plane through (0, 0, 0) normal (0, -1, 0) x (1, 0, 0)
  line L0 (0, -194) -> (0, 0) projected
  line L1 (136, 0) -> (4, 0)
  line L2 (0, -4) -> (0, -190)
  line L3 (4, -194) -> (136, -194)
  line L4 (140, -190) -> (140, -4)
  arc A0 (140, -4) -> (136, 0) centre (136, -4) ccw
  arc A1 (136, -194) -> (140, -190) centre (136, -190) ccw
  arc A2 (0, -190) -> (4, -194) centre (4, -190) ccw
  arc A3 (4, 0) -> (0, -4) centre (4, -4) ccw
  line L5 (140, 0) -> (0, 0)
  line L6 (0, 0) -> (0, -194)
  line L7 (0, -194) -> (140, -194)
  line L8 (140, -194) -> (140, 0)
  point P0 (4, 0)
  dimension "d270" = 4
  constraints: 16 end point, 8 point on circle, 8 tangent, 4 centre point, 4 parallel, 4 point on line, 3 equal radius, 2 horizontal, 2 perpendicular
  measures "d270" radius of A0
extrude "Extrusion15" cut sketch "Skizze16" against normal blind 55 contours L0 A2 L7 | L0 L5 A3 | A1 L8 L7 | L5 L8 A0
sketch "Skizze17" plane through (0, 5, 0) normal (0, 1, 0) x (1, 0, 0)
  line L0 (68, 3) -> (3, 3) projected
  line L1 (3, 3) -> (10, 3)
  line L2 (10, 3) -> (10, 6)
  line L3 (6, 10) -> (3, 10)
  line L4 (3, 10) -> (3, 3)
  line L5 (72, 3) -> (137, 3) projected
  line L6 (137, 3) -> (130, 3)
  line L7 (130, 3) -> (130, 6)
  line L8 (134, 10) -> (137, 10)
  line L9 (137, 10) -> (137, 3)
  line L10 (137, 169.3166) -> (137, 191) projected
  line L11 (137, 191) -> (130, 191)
  line L12 (130, 191) -> (130, 188)
  line L13 (134, 184) -> (137, 184)
  line L14 (137, 184) -> (137, 191)
  line L15 (3, 191) -> (10, 191)
  line L16 (10, 191) -> (10, 188)
  line L17 (6, 184) -> (3, 184)
  line L18 (3, 184) -> (3, 191)
  arc A0 (6, 184) -> (10, 188) centre (6, 188) ccw
  arc A1 (130, 188) -> (134, 184) centre (134, 188) ccw
  arc A2 (134, 10) -> (130, 6) centre (134, 6) ccw
  arc A3 (10, 6) -> (6, 10) centre (6, 6) ccw
  point P0 (0, 0)
  point P1 (10, 10)
  point P2 (130, 10)
  point P3 (130, 184)
  point P4 (10, 184)
  point P5 (10, 3)
  dimension "d273" = 7
  dimension "d274" = 7
  dimension "d275" = 7
  dimension "d276" = 7
  dimension "d277" = 7
  dimension "d278" = 7
  dimension "d279" = 7
  dimension "d280" = 7
  dimension "d283" = 4
  dimension "d285" = 4
  constraints: 32 end point, 10 point on line, 8 parallel, 8 point on circle, 8 tangent, 4 centre point, 4 horizontal, 4 perpendicular, 2 equal radius
  measures "d273" distance of L3.end point (10, 10)
  measures "d274" distance of point (10, 10) L1.end
  measures "d275" distance of point (130, 10) L8.end
  measures "d276" distance of L6.end point (130, 10)
  measures "d277" distance of L13.end point (130, 184)
  measures "d278" distance of point (130, 184) L11.end
  measures "d279" distance of point (10, 184) L17.end
  measures "d280" distance of L15.end point (10, 184)
  measures "d283" radius of A0
  measures "d285" radius of A3
extrude "Extrusion16" add sketch "Skizze17" along normal blind 45
sketch "Skizze18" plane through (0, 50, 0) normal (0, 1, 0) x (1, 0, 0)
  circle A0 centre (5, 5) radius 2.25
  line L0 (0, 190) -> (0, 4) projected
  line L1 (4, 0) -> (136, 0) projected
  circle A1 centre (135, 5) radius 2.25
  circle A2 centre (135, 189) radius 2.25
  circle A3 centre (5, 189) radius 2.25
  line L2 (136, 194) -> (4, 194) projected
  line L3 (140, 4) -> (140, 190) projected
  point P0 (0, 0)
  dimension "d284" = 4.5
  dimension "d286" = 5
  dimension "d287" = 5
  dimension "d288" = 4.5
  dimension "d289" = 4.5
  dimension "d290" = 4.5
  dimension "d291" = 5
  dimension "d292" = 5
  dimension "d293" = 5
  dimension "d294" = 5
  dimension "d295" = 5
  dimension "d296" = 5
  constraints: 4 centre point
  measures "d284" diameter of A0
  measures "d286" distance from line of L0 A0.centre
  measures "d287" distance from line of L1 A0.centre
  measures "d288" diameter of A1
  measures "d289" diameter of A2
  measures "d290" diameter of A3
  measures "d291" distance from line of L0 A3.centre
  measures "d292" distance from line of L2 A3.centre
  measures "d293" distance from line of L2 A2.centre
  measures "d294" distance from line of L3 A2.centre
  measures "d295" distance from line of L1 A1.centre
  measures "d296" distance from line of L3 A1.centre
extrude "Extrusion17" cut sketch "Skizze18" against normal blind 15
sketch "Skizze21" plane through (0, 5, 0) normal (0, 1, 0) x (1, 0, 0)
  line L0 (136, 194) -> (4, 194) projected
  line L1 (4, 0) -> (136, 0) projected
  line L2 (0, 190) -> (0, 4) projected
  point P0 (0, 0)
  point P1 (55, 18)
  point P2 (85, 18)
  point P3 (55, 176)
  point P4 (85, 176)
  dimension "d353" = 30
  dimension "d354" = 30
  dimension "d355" = 18
  dimension "d356" = 18
  dimension "d357" = 18
  dimension "d358" = 18
  dimension "d359" = 55
  dimension "d360" = 55
  measures "d353" distance of point (85, 18) point (55, 18)
  measures "d354" distance of point (85, 176) point (55, 176)
  measures "d355" distance from line of L0 point (55, 176)
  measures "d356" distance from line of L0 point (85, 176)
  measures "d357" distance from line of L1 point (85, 18)
  measures "d358" distance from line of L1 point (55, 18)
  measures "d359" distance from line of point (55, 18) L2
  measures "d360" distance from line of L2 point (55, 176)
hole "Bohrung4" at (55, 5, -18) at (85, 5, -18) at (55, 5, -176) at (85, 5, -176) direction (0, -1, 0) diameter 3 depth 8 tip angle 118 countersink diameter 5.5 countersink angle 90
chamfer "Fase6" distance 2 angle 45 9 edges at (46.5, 27.5, -191) (46.5, 5, -181.4047) (44.5, 5, -181.4896) (44.5, 27.5, -191) (93.5, 5, -181) (94.5, 5, -171) (95.5, 5, -181) (95.5, 27.5, -191) (93.5, 27.5, -191)
chamfer "Fase7" distance 2 angle 45 5 edges at (68, 27.5, -3) (68, 5, -13) (70, 5, -23) (72, 5, -13) (72, 27.5, -3)
sketch "Skizze22" plane through (3, 5, -33) normal (0, 0, 1) x (1, 0, 0)
  line L0 (0, 0) -> (0, 45) projected
  line L1 (25, 0) -> (0, 0) projected
  line L2 (0, 45) -> (25, 0)
  line L3 (0, 45) -> (25, 45) projected
  line L4 (25, 0) -> (25, 45)
  line L5 (25, 45) -> (0, 45)
  point P0 (-3, -5)
  constraints: 6 end point, 2 perpendicular
extrude "Extrusion19" cut sketch "Skizze22" against normal blind 110 contours L3 L4 L2
chamfer "Fase8" distance 2 angle 45 15 edges at (3, 27.5, -35) (15.5, 5, -35) (15.5, 5, -86) (3, 27.5, -86) (3, 27.5, -137) (15.5, 5, -137) (28, 5, -136) (28, 5, -85) (28, 5, -34) (3, 27.5, -135) (15.5, 5, -135) (15.5, 5, -84) (3, 27.5, -84) (3, 27.5, -33) (15.5, 5, -33)
